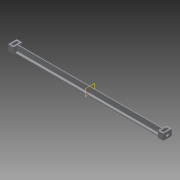
# Autodesk Inventor part: Axle
Saved by Autodesk Inventor 2014 SP1 (Build 180222100, 222)
## iProperties
Created: 2017-01-05
Part Number: Axle
Material: Generic
Document SubType Name: Modeling
Designer: danielsikar
Density: 1 g/cm^3
Appearance: Default
Author: danielsikar
Autodesk Inventor part; units mm, degrees
ref_plane "XZ Plane" through (0, 0, 0) normal (0, 1, 0) x (-1, 0, 0)
ref_plane "XY Plane" through (0, 0, 0) normal (0, 0, 1) x (1, 0, 0)
sketch "Sketch1" plane through (0, 0, 0) normal (0, 0, 1) x (1, 0, 0)
  line L0 (0, 0) -> (200, 0)
  line L1 (200, 0) -> (200, 7)
  line L2 (200, 7) -> (0, 7)
  line L3 (0, 7) -> (0, 0)
  dimension "d0" = 200
  dimension "d1" = 7
  constraints: 8 end point, 2 parallel, 1 horizontal, 1 perpendicular
  measures "d0" distance of L2.end L1.end
  measures "d1" distance of L1.end L0.end
extrude "Extrusion1" add sketch "Sketch1" along normal blind 1.5
sketch "Sketch2" plane through (0, 0, 1.5) normal (0, 0, 1) x (1, 0, 0)
  line L0 (200, 7) -> (0, 7) projected
  line L1 (0, 7) -> (0, 0) projected
  line L2 (0, 4.25) -> (200, 4.25)
  line L3 (200, 4.25) -> (200, 2.75)
  line L4 (200, 2.75) -> (0, 2.75)
  line L5 (0, 2.75) -> (0, 4.25)
  dimension "d4" = 200
  dimension "d5" = 1.5
  dimension "d6" = 2.75
  constraints: 8 end point, 2 parallel, 1 horizontal, 1 perpendicular, 1 point on line
  measures "d4" distance of L3.end L4.end
  measures "d5" distance of L2.end L3.end
  measures "d6" distance between parallel lines of L0 L2
extrude "Extrusion2" add sketch "Sketch2" along normal blind 6.5
sketch "Sketch3" plane through (0, 0, 0) normal (0, 0, -1) x (-1, 0, 0)
  line L0 (-200, 7) -> (0, 7) projected
  line L1 (-200, 9) -> (-193, 9)
  line L2 (-193, 9) -> (-193, -2)
  line L3 (-193, -2) -> (-200, -2)
  line L4 (-200, -2) -> (-200, 9)
  dimension "d9" = 7
  dimension "d10" = 11
  dimension "d11" = 2
  constraints: 8 end point, 2 parallel, 1 horizontal, 1 perpendicular
  measures "d9" distance of L2.end L3.end
  measures "d10" distance of L1.end L2.end
  measures "d11" distance between parallel lines of L1 L0
extrude "Extrusion3" add sketch "Sketch3" against normal up to surface (8 mm away)
sketch "Sketch4" plane through (0, 0, 0) normal (0, 0, -1) x (-1, 0, 0)
  line L0 (-200, 9) -> (-193, 9) projected
  line L1 (-200, -2) -> (-200, 9) projected
  line L2 (-193, -2) -> (-200, -2) projected
  line L3 (-198.25, 7.15) -> (-194.75, 7.15)
  line L4 (-194.75, 7.15) -> (-194.75, -0.15)
  line L5 (-194.75, -0.15) -> (-198.25, -0.15)
  line L6 (-198.25, -0.15) -> (-198.25, 7.15)
  dimension "d14" = 3.5
  dimension "d15" = 7.3
  dimension "d16" = 1.85
  dimension "d17" = 1.85
  dimension "d18" = 1.75
  constraints: 8 end point, 2 parallel, 1 horizontal, 1 perpendicular
  measures "d14" distance of L4.end L5.end
  measures "d15" distance of L3.end L4.end
  measures "d16" distance between parallel lines of L0 L3
  measures "d17" distance between parallel lines of L2 L5
  measures "d18" distance between parallel lines of L1 L6
extrude "Extrusion4" cut sketch "Sketch4" against normal blind 8
sketch "Sketch5" plane through (200, -2, 0) normal (1, 0, 0) x (0, 0, -1)
  circle A0 centre (-4, 5.5) radius 2.1
  point P0 (0, 2)
  dimension "d21" = 4.2
  constraints: 1 centre point
  measures "d21" diameter of A0
ref_plane "Work Plane1" through (100, 0, 0) normal (1, 0, 0) x (0, 1, 0)
extrude "Extrusion5" cut sketch "Sketch5" against normal up to surface (7 mm away)
mirror "Mirror1" about plane through (100, 0, 0) normal (1, 0, 0) of "Extrusion3"
mirror "Mirror2" about plane through (100, 0, 0) normal (1, 0, 0) of "Extrusion5", "Extrusion4"
sketch "Sketch6" plane through (0, 0, 1.5) normal (0, 0, 1) x (1, 0, 0)
  line L0 (7, 7) -> (7, 4.25) projected
  line L1 (7, 4.25) -> (193, 4.25) projected
  line L2 (193, 4.25) -> (193, 7) projected
  line L3 (193, 7) -> (7, 7) projected
  point P0 (0, 0)
extrude "Extrusion6" cut sketch "Sketch6" against normal blind 0.5
sketch "Sketch7" plane through (0, 0, 1.5) normal (0, 0, 1) x (1, 0, 0)
  line L0 (7, 2.75) -> (7, 0) projected
  line L1 (7, 0) -> (193, 0) projected
  line L2 (193, 0) -> (193, 2.75) projected
  line L3 (193, 2.75) -> (7, 2.75) projected
  point P0 (0, 0)
extrude "Extrusion7" cut sketch "Sketch7" against normal blind 0.5
sketch "Sketch8" plane through (193, 4.25, 5.9615) normal (0, 1, 0) x (1, 0, 0)
  line L0 (-186, 4.9615) -> (-186, 3.923) projected
  line L1 (-186, 3.923) -> (-186, 0) projected
  line L2 (-186, 0) -> (-186, -2.0385) projected
  line L3 (0, -2.0385) -> (-186, -2.0385) projected
  line L4 (0, -2.0385) -> (0, 0) projected
  line L5 (0, 0) -> (0, 3.923) projected
  line L6 (0, 3.923) -> (0, 4.9615) projected
  line L7 (0, 4.9615) -> (-186, 4.9615) projected
  point P0 (-193, 5.9615)
extrude "Extrusion8" cut sketch "Sketch8" against normal blind 0.25
sketch "Sketch9" plane through (193, 2.75, 2.0385) normal (0, -1, 0) x (1, 0, 0)
  line L0 (-186, 5.9615) -> (-186, 3.923) projected
  line L1 (-186, 3.923) -> (-186, 0) projected
  line L2 (-186, 0) -> (-186, -1.0385) projected
  line L3 (-186, -1.0385) -> (0, -1.0385) projected
  line L4 (0, -1.0385) -> (0, 0) projected
  line L5 (0, 0) -> (0, 3.923) projected
  line L6 (0, 3.923) -> (0, 5.9615) projected
  line L7 (-186, 5.9615) -> (0, 5.9615) projected
  point P0 (-193, -2.0385)
extrude "Extrusion9" cut sketch "Sketch9" against normal blind 0.25
sketch "Sketch10" plane through (194.75, -0.15, 0) normal (1, 0, 0) x (0, 0, -1)
  circle A0 centre (-4, 3.65) radius 2.1 projected
  point P0 (0, 0.15)
extrude "Extrusion10" add sketch "Sketch10" against normal up to surface (1.75 mm away)
mirror "Mirror3" about plane through (100, 0, 0) normal (1, 0, 0) of "Extrusion10"
body "Solid1"
